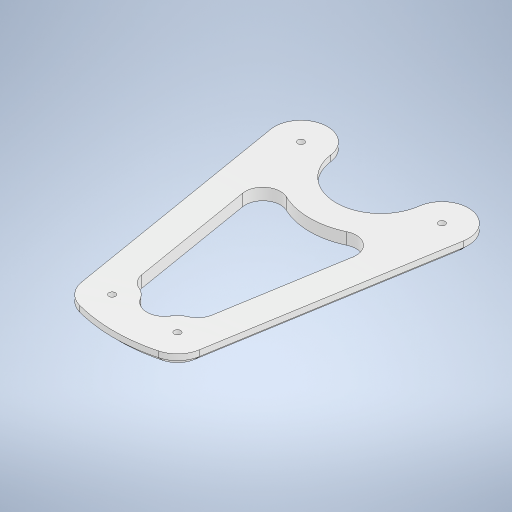
# Autodesk Inventor part: Upright - Lower
Saved by Autodesk Inventor 2023.2 (Build 272271000, 271)
## iProperties
Created: 2023-10-14
Part Number: Upright - Lower
Material: UHMW, White
Document SubType Name: Modeling
Designer: Nathan Cai
Mass: 87.7146 g
Surface Area: 154.327 cm^2
Volume: 32.4869 cm^3
Density: 0.94 g/cm^3
Appearance: Smooth - White
Author: Nathan Cai
Autodesk Inventor part; units mm, degrees
ref_plane "YZ Plane" through (0, 0, 0) normal (1, 0, 0) x (0, 1, 0)
ref_plane "XZ Plane" through (0, 0, 0) normal (0, 1, 0) x (-1, 0, 0)
ref_plane "XY Plane" through (0, 0, 0) normal (0, 0, 1) x (1, 0, 0)
sketch "Sketch1" plane through (0, 0, 0) normal (0, 1, 0) x (-1, 0, 0)
  circle A0 centre (0, 0) radius 38.1 construction
  line L0 (38.1, 0) -> (-38.1, 0) construction
  circle A1 centre (38.1, 0) radius 1.7526
  circle A2 centre (-38.1, 0) radius 1.7526
  circle A3 centre (38.1, 0) radius 7.9375 construction
  circle A4 centre (-38.1, 0) radius 7.9375 construction
  line L1 (0, 0) -> (0, -38.1) construction
  circle A5 centre (0, 56.6406) radius 76.2 construction
  circle A6 centre (-17.6676, 122.5771) radius 7.9375 construction
  circle A7 centre (-17.6676, 122.5771) radius 1.7526
  circle A8 centre (-38.1, 0) radius 11.1125
  circle A9 centre (38.1, 0) radius 11.1125
  circle A10 centre (-17.6676, 122.5771) radius 11.1125
  line L2 (0, 56.6406) -> (0, 132.8406) construction
  line L3 (0, 56.6406) -> (-17.6676, 122.5771) construction
  line L4 (-49.0613, 1.8271) -> (-28.6289, 124.4043)
  line L5 (-38.1, 0) -> (-17.6676, 122.5771) construction
  circle A11 centre (17.6676, 122.5771) radius 7.9375 construction
  circle A12 centre (17.6676, 122.5771) radius 1.7526
  circle A13 centre (17.6676, 122.5771) radius 11.1125
  line L6 (49.0613, 1.8271) -> (28.6289, 124.4043)
  line L7 (38.1, 0) -> (17.6676, 122.5771) construction
  arc A14 (20.5438, 133.311) -> (-20.5438, 133.311) centre (0, 56.6406) ccw
  arc A15 (-44.3023, -9.2206) -> (44.3023, -9.2206) centre (0, 56.6406) ccw
  arc A16 (17.6676, 122.5771) -> (-17.6676, 122.5771) centre (0, 56.6406) ccw
  arc A17 (-38.1, 0) -> (38.1, 0) centre (0, 56.6406) ccw
  line L8 (-34.7257, 10.5878) -> (-17.9101, 111.4673)
  line L9 (34.7257, 10.5878) -> (17.9101, 111.4673)
  circle A18 centre (0, 0) radius 19.5594
  arc A19 (27.0858, -1.4751) -> (-27.0858, -1.4751) centre (0, -5.1027) ccw
  circle A20 centre (0, 0) radius 22.225 construction
  arc A21 (38.1, 0) -> (-38.1, 0) centre (0, -5.1027) ccw
  point P0 (49.0613, 1.8271)
  point P1 (6.7353, 124.57)
  point P2 (17.9101, 111.4673)
  point P3 (28.4052, -5.4312)
  point P4 (-28.4052, -5.4312)
  point P5 (-6.7353, 124.57)
  point P6 (17.1322, -9.437)
  point P7 (-17.1322, -9.437)
  point P8 (34.5232, 11.8029)
  point P9 (-34.5232, 11.8029)
  dimension "d5" = 152.4
  dimension "d0" = 76.2
  dimension "d1" = 3.5052
  dimension "d2" = 3.5052
  dimension "d3" = 15.875
  dimension "d4" = 15.875
  dimension "d8" = 15.875
  dimension "d9" = 3.5052
  dimension "d11" = 15
  dimension "d12" = 79.375
  dimension "d13" = 79.375
  dimension "d17" = 11.1125
  dimension "d18" = 11.1125
  dimension "d20" = 12.7
  dimension "d21" = 44.45
  dimension "d22" = 11.1125
  constraints: 26 point on circle, 21 centre point, 20 end point, 14 coincident, 8 symmetric about line, 8 tangent, 1 horizontal, 1 midpoint, 1 parallel, 1 perpendicular, 1 point on line, 1 vertical, 1 vertical alignment, 8 other
  measures "d0" diameter of A0
  measures "d1" diameter of A1
  measures "d2" diameter of A2
  measures "d3" diameter of A3
  measures "d4" diameter of A4
  measures "d8" diameter of A6
  measures "d9" diameter of A7
  measures "d11" angle of L2 L3
  measures "d12" radius of A15
  measures "d13" radius of A14
  measures "d17" radial gap between concentric circles of A14 A16
  measures "d18" radial gap between concentric circles of A15 A17
  measures "d20" distance between parallel lines of L4 L8
  measures "d21" diameter of A20
  measures "d22" radial gap between concentric circles of A19 A21
extrude "Extrusion1" add sketch "Sketch1" along normal blind 6.35 contours A1 A21 A9 A17 | A1 A17 A9 A21 | A21 L9 A13 L6 A9 | A9 L9 A21 | A9 A19 A8 L8 A21 L9 | A13 | A21 A8 L4 A10 L8 | L8 A8 A21 | A8 A17 A2 A21 | A8 A21 A2 A17 | A13 A16 A10 A14 | A10
fillet "Fillet1" radius 9.525 6 edges at (17.9101, 3.175, 111.4673) (6.7353, 3.175, 124.57) (-6.7353, 3.175, 124.57) (-17.9101, 3.175, 111.4673) (-34.5232, 3.175, 11.8029) (34.5232, 3.175, 11.8029)
thicken "Thicken1" operation add thickness 3.175 both sides no extend neighbours no toward (0.9863902, 0, 0.1644213) faces at (35.4397, 2.1167, 83.5452) (39.303, 4.2333, -11.0472) (25.605, 4.2333, 130.3544) (8.5829, 4.2333, 20.8422) (-3.4623, 4.2333, 135.9401) (-49.1735, 4.2333, 0.9301) (-25.605, 4.2333, 130.3544) (-42.2505, 2.1167, 42.6862)
chamfer "Chamfer1" distance 3.175 angle 45 8 edges at (41.9769, 0, 63.6377) (40.2231, 0, -14.1289) (0, 0, 19.05) (-40.2231, 0, -14.1289) (-41.9769, 0, 63.6377) (-28.2466, 0, 132.1802) (0, 0, 139.1906) (28.2466, 0, 132.1802)
chamfer "Chamfer2" distance 3.175 angle 45 4 edges at (19.4202, 0, 122.5771) (-15.915, 0, 122.5771) (39.8526, 0, 0) (-36.3474, 0, 0)
equation "\"d1\" = d2"
equation "\"d9\" = d2"
equation "\"d13\" = d12"
body "Solid1"
